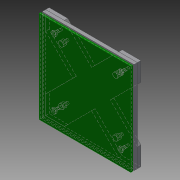
# Autodesk Inventor part: crane
Saved by Autodesk Inventor 2014 (Build 180170000, 170)
## iProperties
Created: 2015-03-06
Part Number: crane
Material: Generic
Document SubType Name: Modeling
Designer: cruiser
Density: 1 g/cm^3
Appearance: Default
Author: cruiser
Autodesk Inventor part; units mm, degrees
ref_plane "YZ Plane" through (0, 0, 0) normal (1, 0, 0) x (0, 1, 0)
ref_plane "XZ Plane" through (0, 0, 0) normal (0, 1, 0) x (-1, 0, 0)
ref_plane "XY Plane" through (0, 0, 0) normal (0, 0, 1) x (1, 0, 0)
sketch "Sketch1" plane through (0, 0, 0) normal (0, 1, 0) x (-1, 0, 0)
  line L0 (73.5, -73.5) -> (-73.5, -73.5)
  line L1 (-73.5, -73.5) -> (-73.5, 73.5)
  line L2 (-73.5, 73.5) -> (73.5, 73.5)
  line L3 (73.5, 73.5) -> (73.5, -73.5)
  line L4 (73.5, -73.5) -> (-73.5, 73.5) construction
  line L5 (-73.5, -73.5) -> (73.5, 73.5) construction
  point P0 (0, 0)
  dimension "d0" = 147
  dimension "d1" = 147
  constraints: 12 end point, 2 midpoint, 2 parallel, 1 horizontal, 1 perpendicular
  measures "d0" distance of L0.end L1.end
  measures "d1" distance of L1.end L2.end
extrude "Extrusion1" add sketch "Sketch1" along normal blind 5.6
sketch "Sketch9" plane through (0, 5.6, 0) normal (0, 1, 0) x (1, 0, 0)
  line L0 (73.5, 73.5) -> (-73.5, 73.5) projected
  line L1 (-73.5, 73.5) -> (-73.5, -73.5) projected
  line L2 (-73.5, -73.5) -> (73.5, -73.5) projected
  line L3 (73.5, -73.5) -> (73.5, 73.5) projected
  circle A0 centre (-43.5, 43.5) radius 2
  circle A1 centre (43.5, 43.5) radius 2
  circle A2 centre (-43.5, -43.5) radius 2
  circle A3 centre (43.5, -43.5) radius 2
  circle A4 centre (-53.5, 53.5) radius 1.65
  circle A5 centre (53.5, 53.5) radius 1.65
  circle A6 centre (-53.5, -53.5) radius 1.65
  circle A7 centre (53.5, -53.5) radius 1.65
  point P0 (0, 0)
  dimension "d56" = 4
  dimension "d57" = 30
  dimension "d58" = 30
  dimension "d61" = 87
  dimension "d64" = 87
  dimension "d76" = 3.3
  dimension "d77" = 20
  dimension "d78" = 20
  dimension "d81" = 107
  dimension "d84" = 107
  constraints: 8 centre point, 2 horizontal, 2 vertical, 12 other
  measures "d56" diameter of A0
  measures "d57" distance from line of L1 A0.centre
  measures "d58" distance from line of L0 A0.centre
  measures "d61" distance of A0.centre A1.centre
  measures "d64" distance of A0.centre A2.centre
  measures "d76" diameter of A4
  measures "d77" distance from line of L0 A4.centre
  measures "d78" distance from line of L1 A4.centre
  measures "d81" distance of A4.centre A5.centre
  measures "d84" distance of A4.centre A6.centre
extrude "Extrusion8" add sketch "Sketch9" along normal blind 5.6 separate body
sketch "Sketch2" plane through (0, 0, 0) normal (0, -1, 0) x (1, 0, 0)
  line L0 (73.5, -73.5) -> (73.5, 73.5) projected
  line L1 (73.5, 73.5) -> (-73.5, 73.5) projected
  line L2 (-73.5, 73.5) -> (-73.5, -73.5) projected
  circle A0 centre (-53.5, 53.5) radius 2
  circle A1 centre (53.5, 53.5) radius 2
  circle A2 centre (-53.5, -53.5) radius 2
  circle A3 centre (53.5, -53.5) radius 2
  point P0 (0, 0)
  dimension "d4" = 4
  dimension "d5" = 20
  dimension "d6" = 20
  dimension "d9" = 107
  dimension "d12" = 107
  constraints: 4 centre point, 1 horizontal, 1 vertical, 6 other
  measures "d4" diameter of A0
  measures "d5" distance from line of L1 A0.centre
  measures "d6" distance from line of L2 A0.centre
  measures "d9" distance of A0.centre A1.centre
  measures "d12" distance of A0.centre A2.centre
extrude "Extrusion2" cut sketch "Sketch2" against normal blind 107 bodies 1
sketch "Sketch3" plane through (0, 0, 0) normal (0, -1, 0) x (1, 0, 0)
  circle A0 centre (-53.5, -53.5) radius 2 projected
  circle A1 centre (-53.5, 53.5) radius 2 projected
  circle A2 centre (53.5, 53.5) radius 2 projected
  circle A3 centre (53.5, -53.5) radius 2 projected
  line L0 (73.5, 73.5) -> (-73.5, 73.5) projected
  line L1 (-73.5, 73.5) -> (-73.5, -73.5) projected
  circle A4 centre (-53.5, 53.5) radius 4
  circle A5 centre (53.5, 53.5) radius 4
  circle A6 centre (53.5, -53.5) radius 4
  circle A7 centre (-53.5, -53.5) radius 4
  line L2 (71.5, -71.5) -> (-71.5, -71.5)
  line L3 (-71.5, -71.5) -> (-71.5, 71.5)
  line L4 (-71.5, 71.5) -> (71.5, 71.5)
  line L5 (71.5, 71.5) -> (71.5, -71.5)
  line L6 (71.5, -71.5) -> (-71.5, 71.5) construction
  line L7 (-71.5, -71.5) -> (71.5, 71.5) construction
  point P0 (0, 0)
  dimension "d17" = 8
  dimension "d18" = 8
  dimension "d19" = 8
  dimension "d20" = 8
  dimension "d21" = 2
  dimension "d22" = 2
  constraints: 12 end point, 4 centre point, 4 coincident, 2 midpoint, 2 parallel, 1 horizontal, 1 perpendicular
  measures "d17" diameter of A4
  measures "d18" diameter of A5
  measures "d19" diameter of A7
  measures "d20" diameter of A6
  measures "d21" distance between parallel lines of L0 L4
  measures "d22" distance between parallel lines of L1 L3
extrude "Extrusion3" add sketch "Sketch3" along normal blind 2 separate body contours L2 L3 L4 L5
sketch "Sketch4" plane through (0, -2, 0) normal (0, -1, 0) x (1, 0, 0)
  circle A0 centre (-53.5, -53.5) radius 4 projected
  circle A1 centre (53.5, -53.5) radius 4 projected
  circle A2 centre (53.5, 53.5) radius 4 projected
  circle A3 centre (-53.5, 53.5) radius 4 projected
  line L0 (-71.5, -71.5) -> (71.5, -71.5) projected
  line L1 (71.5, -71.5) -> (71.5, 71.5) projected
  line L2 (71.5, 71.5) -> (-71.5, 71.5) projected
  line L3 (-71.5, 71.5) -> (-71.5, -71.5) projected
  line L4 (73.5, -73.5) -> (-73.5, -73.5)
  line L5 (-73.5, -73.5) -> (-73.5, 73.5)
  line L6 (-73.5, 73.5) -> (73.5, 73.5)
  line L7 (73.5, 73.5) -> (73.5, -73.5)
  line L8 (73.5, -73.5) -> (-73.5, 73.5) construction
  line L9 (-73.5, -73.5) -> (73.5, 73.5) construction
  point P0 (0, 0)
  dimension "d25" = 147
  dimension "d26" = 147
  constraints: 12 end point, 2 midpoint, 2 parallel, 1 horizontal, 1 perpendicular
  measures "d25" distance of L4.end L5.end
  measures "d26" distance of L5.end L6.end
extrude "Extrusion4" add sketch "Sketch4" along normal blind 3 separate body contours A0 | A1 | A2 | A3 | L3 L2 L1 L0 | L4 L5 L6 L7
sketch "Sketch8" plane through (0, 5.6, 0) normal (0, 1, 0) x (1, 0, 0)
  line L0 (73.5, 73.5) -> (-73.5, 73.5) projected
  line L1 (-73.5, 73.5) -> (-73.5, -73.5) projected
  circle A0 centre (-43.5, 43.5) radius 4
  circle A1 centre (43.5, 43.5) radius 4
  circle A2 centre (-43.5, -43.5) radius 4
  circle A3 centre (43.5, -43.5) radius 4
  point P0 (0, 0)
  dimension "d43" = 30
  dimension "d44" = 30
  dimension "d45" = 8
  dimension "d48" = 87
  dimension "d51" = 87
  constraints: 4 centre point, 1 horizontal, 1 vertical, 6 other
  measures "d43" distance from line of L1 A0.centre
  measures "d44" distance from line of L0 A0.centre
  measures "d45" diameter of A0
  measures "d48" distance of A0.centre A1.centre
  measures "d51" distance of A0.centre A2.centre
extrude "Extrusion7" cut sketch "Sketch8" against normal up to next bodies 1
sketch "Sketch6" plane through (0, 5.6, 0) normal (0, 1, 0) x (1, 0, 0)
  line L0 (73.5, 73.5) -> (-73.5, 73.5) projected
  line L1 (-73.5, 73.5) -> (-73.5, -73.5) projected
  line L2 (-73.5, -73.5) -> (73.5, -73.5) projected
  line L3 (73.5, -73.5) -> (73.5, 73.5) projected
  line L4 (33.5, -33.5) -> (-33.5, -33.5)
  line L5 (-33.5, -33.5) -> (-33.5, 33.5)
  line L6 (-33.5, 33.5) -> (33.5, 33.5)
  line L7 (33.5, 33.5) -> (33.5, -33.5)
  line L8 (33.5, -33.5) -> (-33.5, 33.5) construction
  line L9 (-33.5, -33.5) -> (33.5, 33.5) construction
  line L10 (0, 33.5) -> (40, 73.5)
  line L11 (0, 33.5) -> (56.5685, 33.5) construction
  line L12 (-33.5, 0) -> (-73.5, 40)
  line L13 (-33.5, 0) -> (-73.5, -40)
  line L14 (0, -33.5) -> (-40, -73.5)
  line L15 (0, -33.5) -> (40, -73.5)
  line L16 (33.5, 0) -> (73.5, -40)
  line L17 (33.5, 0) -> (73.5, 40)
  line L18 (0, 33.5) -> (-40, 73.5)
  point P0 (0, 0)
  dimension "d32" = 40
  dimension "d33" = 40
  dimension "d34" = 45
  dimension "d35" = 45
  constraints: 30 end point, 8 point on line, 6 midpoint, 5 perpendicular, 4 parallel, 2 horizontal, 1 equal length
  measures "d32" distance between parallel lines of L0 L6
  measures "d33" distance between parallel lines of L3 L7
  measures "d34" angle of L11 L10
  measures "d35" angle of L6 L18
extrude "Extrusion5" [suppressed]
sketch "Sketch7" plane through (0, -2, 0) normal (0, -1, 0) x (1, 0, 0)
  line L0 (-71.5, -71.5) -> (71.5, -71.5) projected
  line L1 (71.5, -71.5) -> (71.5, 71.5) projected
  line L2 (71.5, 71.5) -> (-71.5, 71.5) projected
  line L3 (-71.5, 71.5) -> (-71.5, -71.5) projected
  line L4 (29.5, -29.5) -> (-29.5, -29.5)
  line L5 (-29.5, -29.5) -> (-29.5, 29.5)
  line L6 (-29.5, 29.5) -> (29.5, 29.5)
  line L7 (29.5, 29.5) -> (29.5, -29.5)
  line L8 (29.5, -29.5) -> (-29.5, 29.5) construction
  line L9 (-29.5, -29.5) -> (29.5, 29.5) construction
  line L10 (0, 29.5) -> (42, 71.5)
  line L11 (0, 29.5) -> (59.397, 29.5) construction
  line L12 (0, 29.5) -> (-42, 71.5)
  line L13 (-29.5, 0) -> (-71.5, 42)
  line L14 (-29.5, 0) -> (-71.5, -42)
  line L15 (0, -29.5) -> (-42, -71.5)
  line L16 (0, -29.5) -> (42, -71.5)
  line L17 (29.5, 0) -> (71.5, 42)
  line L18 (29.5, 0) -> (71.5, -42)
  point P0 (0, 0)
  dimension "d38" = 42
  dimension "d39" = 42
  dimension "d40" = 45
  constraints: 30 end point, 8 point on line, 6 midpoint, 6 perpendicular, 4 parallel, 2 horizontal, 1 equal length
  measures "d38" distance between parallel lines of L1 L7
  measures "d39" distance between parallel lines of L2 L6
  measures "d40" angle of L11 L10
extrude "Extrusion6" [suppressed]
sketch "Sketch10" plane through (0, 11.2, 0) normal (0, 1, 0) x (1, 0, 0)
  line L0 (73.5, 73.5) -> (-73.5, 73.5) projected
  line L1 (0, 30) -> (-43.5, 73.5)
  line L2 (-43.5, 73.5) -> (0, 117)
  line L3 (0, 117) -> (43.5, 73.5)
  line L4 (43.5, 73.5) -> (0, 30)
  line L5 (-43.5, 73.5) -> (43.5, 73.5)
  line L6 (-30, 0) -> (-73.5, -43.5)
  line L7 (-73.5, 43.5) -> (-30, 0)
  line L8 (-73.5, -43.5) -> (-73.5, 43.5)
  line L9 (0, -30) -> (43.5, -73.5)
  line L10 (-43.5, -73.5) -> (0, -30)
  line L11 (43.5, -73.5) -> (-43.5, -73.5)
  line L12 (30, 0) -> (73.5, 43.5)
  line L13 (73.5, -43.5) -> (30, 0)
  line L14 (73.5, 43.5) -> (73.5, -43.5)
  point P0 (0, 0)
  point P1 (0, 73.5)
  point P2 (-73.5, 0)
  point P3 (0, -73.5)
  point P4 (73.5, 0)
  dimension "d69" = 30
  dimension "d72" = 360
  constraints: 28 end point, 1 collinear, 1 midpoint, 1 point on line, 38 other
  measures "d69" distance of point (0, 0) L1.start
extrude "Extrusion9" cut sketch "Sketch10" against normal up to next contours L4 L1 L0 | L6 L8 L7 | L9 L11 L10 | L12 L14 L13 bodies 2
sketch "Sketch11" plane through (0, -5, 0) normal (0, -1, 0) x (1, 0, 0)
  line L0 (-73.5, -73.5) -> (73.5, -73.5) projected
  line L1 (73.5, -73.5) -> (73.5, 73.5) projected
  line L2 (73.5, 73.5) -> (-73.5, 73.5) projected
  line L3 (-73.5, 73.5) -> (-73.5, -73.5) projected
  line L4 (-75.5, -75.5) -> (75.5, -75.5)
  line L5 (75.5, -75.5) -> (75.5, 75.5)
  line L6 (75.5, 75.5) -> (-75.5, 75.5)
  line L7 (-75.5, 75.5) -> (-75.5, -75.5)
  line L8 (-75.5, -75.5) -> (75.5, 75.5) construction
  line L9 (75.5, -75.5) -> (-75.5, 75.5) construction
  circle A0 centre (-65.5, 65.5) radius 10
  line L10 (-75.5, 75.5) -> (-65.5, 75.5)
  line L11 (-65.5, 75.5) -> (-65.5, 55.5)
  line L12 (-65.5, 55.5) -> (-75.5, 55.5)
  line L13 (-75.5, 55.5) -> (-75.5, 75.5)
  line L14 (-75.5, 75.5) -> (-55.5, 75.5)
  line L15 (-55.5, 75.5) -> (-55.5, 65.5)
  line L16 (-55.5, 65.5) -> (-75.5, 65.5)
  line L17 (-75.5, 65.5) -> (-75.5, 75.5)
  point P0 (0, 0)
  dimension "d87" = 151
  dimension "d88" = 151
  dimension "d89" = 20
  dimension "d90" = 10
  dimension "d91" = 10
  dimension "d92" = 10
  dimension "d93" = 10
  constraints: 28 end point, 6 parallel, 3 horizontal, 3 perpendicular, 2 midpoint, 2 point on circle, 1 centre point
  measures "d87" distance of L6.end L5.end
  measures "d88" distance of L5.end L4.end
  measures "d89" diameter of A0
  measures "d90" distance from line of L7 A0.centre
  measures "d91" distance from line of L6 A0.centre
  measures "d92" distance of L14.end L15.end
  measures "d93" distance of L11.end L12.end
equation "\"d0\" = bed_y"
equation "\"d1\" = bed_x"
equation "\"t_backing\" = thick_acrylic"
equation "\"d56\" = brass_insert_drill"
equation "\"d57\" = spring_border"
equation "\"d58\" = spring_border"
equation "\"d61\" = bed_x - 2 * spring_border"
equation "\"d64\" = bed_y - 2 * spring_border"
equation "\"d77\" = bed_clamp_border"
equation "\"d78\" = bed_clamp_border"
equation "\"d81\" = bed_x - 2 * bed_clamp_border"
equation "\"d84\" = bed_y - 2 * bed_clamp_border"
equation "\"t_interface\" = thick_acrylic"
equation "\"d4\" = brass_insert_drill"
equation "\"d5\" = bed_clamp_border"
equation "\"d6\" = bed_clamp_border"
equation "\"d9\" = bed_x - 2 * bed_clamp_border"
equation "\"d12\" = bed_x - 2 * bed_clamp_border"
equation "\"d15\" = d9"
equation "\"d17\" = brass_keep_out"
equation "\"d18\" = brass_keep_out"
equation "\"d19\" = brass_keep_out"
equation "\"d20\" = brass_keep_out"
equation "\"d21\" = tape_keep_out"
equation "\"d22\" = tape_keep_out"
equation "\"d23\" = tape_thickness"
equation "\"d25\" = bed_y"
equation "\"d26\" = bed_x"
equation "\"t_bed\" = thin_acrylic"
equation "\"d43\" = spring_border"
equation "\"d44\" = spring_border"
equation "\"d48\" = bed_x - 2 * spring_border"
equation "\"d51\" = bed_y - 2 * spring_border"
equation "\"d32\" = bed_cutout"
equation "\"d33\" = bed_cutout"
equation "\"d38\" = bed_cutout + tape_keep_out"
equation "\"d39\" = bed_cutout + tape_keep_out"
equation "\"d74\" = thick_acrylic"
equation "\"d87\" = reservoir_x"
equation "\"d88\" = reservoir_y"
equation "\"wood_thickness\" = 6.4"
equation "\"m3_diameter\" = 3.15"
equation "\"m5_diameter\" = 5.25"
equation "\"stepper_screw_space\" = 35"
equation "\"stepper_shaft_diameter\" = 5"
equation "\"stepper_body_diameter\" = 28"
equation "\"laser_body_diameter\" = 12"
equation "\"thick_acrylic\" = 5.6"
equation "\"carrier_y\" = 181"
equation "\"reservoir_x\" = 151"
equation "\"reservoir_y\" = 151"
equation "\"thin_acrylic\" = 3"
equation "\"linear_bearing_spacing\" = 207"
equation "\"motor_spacing\" = 287"
equation "\"tray_boarder\" = 15"
equation "\"tray_x\" = 181"
equation "\"tray_y\" = 181"
equation "\"bed_x\" = 147"
equation "\"bed_y\" = 147"
equation "\"spring_boarder\" = 15"
equation "\"brass_insert_drill\" = 4"
equation "\"brass_keep_out\" = 8"
equation "\"tape_keep_out\" = 2"
equation "\"tape_thickness\" = 2"
equation "\"bed_cutout\" = 40"
equation "\"spring_border\" = 30"
equation "\"crane_x\" = 245.2"
equation "\"crane_z\" = 25"
equation "\"z_min_from_center\" = 72.6"
equation "\"printer_z\" = 289"
equation "\"bed_clamp_border\" = 20"
equation "\"linear_bearing_z\" = 304.8"
equation "\"threaded_rod_z\" = 203.2"
equation "\"carrier_z\" = 258.6"
equation "\"carrier_z2\" = 283.6"
equation "\"window_z\" = 185"
equation "\"frame_tilt\" = 1deg"
equation "\"lcd_y\" = 25"
equation "\"lcd_x\" = 72"
equation "\"clear_acrylic\" = 3"
equation "\"laser_z\" = 18"
equation "\"laser_diameter\" = 12"
equation "\"laser_y_offset\" = 19.4"
equation "\"subframe_y_offset\" = 27.5"
equation "\"laser_y\" = 35"
equation "\"frame_top_z\" = 295"
equation "\"frame_y\" = 66.2"
equation "\"frame_bottom_z\" = 225"
equation "\"t_frame\" = 6.4"
equation "\"frame_border\" = 39.5"
equation "\"t_carrier\" = 5.6"
equation "\"t_tray\" = 3"
equation "\"tray_border\" = 15"
equation "\"t_wall\" = 5.6"
equation "\"galvo_frame_z\" = 65"
equation "\"galvo_frame_x\" = 66"
equation "\"t_galvo_frame\" = 5.6"
equation "\"galvo_frame_y_offset\" = 27.5"
equation "\"m4_diameter\" = 4.2"
equation "\"laser_z_offset\" = 55"
equation "\"window_y\" = 51"
equation "\"t_window\" = 3"
equation "\"drawer_z\" = 206.4"
equation "\"drawer_y\" = 51"
equation "\"drawer_x\" = 181"
equation "\"frame_foot_z\" = 49.5"
equation "\"drawer_z_from_bottom\" = 25"
equation "\"end_stop_offset_x\" = 64"
equation "\"t_crane\" = 5.6"
equation "\"end_stop_spacing\" = 9.5"
equation "\"thumb_nut_offset_y\" = 13.6"
equation "\"thumb_nut_diameter\" = 14"
equation "\"frame_foot_extension\" = 4"
